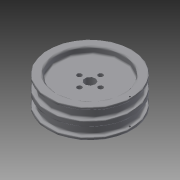
# Autodesk Inventor part: Spool
Saved by Autodesk Inventor 2014 SP2 (Build 180246200, 246)
## iProperties
Created: 2014-09-14
Part Number: Spool
Material: Generic
Document SubType Name: Modeling
Designer: Allison
Density: 1 g/cm^3
Appearance: Default
Author: Allison
Autodesk Inventor part; units mm, degrees
ref_plane "YZ Plane" through (0, 0, 0) normal (1, 0, 0) x (0, 1, 0)
ref_plane "XZ Plane" through (0, 0, 0) normal (0, 1, 0) x (-1, 0, 0)
ref_plane "XY Plane" through (0, 0, 0) normal (0, 0, 1) x (1, 0, 0)
sketch "Sketch1" plane through (0, 0, 0) normal (0, 1, 0) x (-1, 0, 0)
  circle A0 centre (0, 0) radius 31.75
  dimension "d0" = 63.5
  constraints: 1 centre point, 1 coincident
  measures "d0" diameter of A0
sketch "Sketch2" plane through (0, 0, 0) normal (1, 0, 0) x (0, 1, 0)
  line L0 (0, -31.75) -> (0, 31.75) projected
  line L1 (-3.6603, 0) -> (9.0397, 0)
  line L2 (9.0397, 0) -> (9.0397, 31.75)
  line L3 (-3.6603, 31.75) -> (-3.6603, 0)
  line L4 (-3.6603, 31.75) -> (-1.7553, 31.75)
  line L5 (-1.7553, 31.75) -> (-1.7553, 29.21)
  line L6 (9.0397, 31.75) -> (7.1347, 31.75)
  line L7 (7.1347, 31.75) -> (7.1347, 29.21)
  line L8 (7.1347, 29.21) -> (-1.7553, 29.21)
  line L9 (-3.6603, 0) -> (-3.6603, 4.0132)
  line L10 (-3.6603, 4.0132) -> (9.0397, 4.0132)
  line L11 (9.0397, 4.0132) -> (9.0397, 0)
  line L12 (9.0397, 0) -> (-3.6603, 0)
  line L13 (-3.6603, 0) -> (-3.6603, 4.0132)
  point P0 (0, 0)
  dimension "d1" = 12.7
  dimension "d2" = 1.905
  dimension "d5" = 1.905
  dimension "d6" = 31.75
  dimension "d7" = 4.0132
  constraints: 26 end point, 3 parallel, 2 horizontal, 2 perpendicular, 1 point on line
  measures "d1" distance of L3.start L2.end
  measures "d2" distance of L3.start L4.end
  measures "d5" distance of L2.end L6.end
  measures "d6" distance of L3.start L1.start
  measures "d7" distance of L1.start L9.end
revolve "Revolution1" add sketch "Sketch2" angle 360 about axis through (0, -3.6603, 0) along (0, 1, 0) contours L10 L3 L4 L5 L8 L0 | L0 L8 L7 L6 L2 L10
sketch "Sketch3" plane through (0, -3.6603, 0) normal (0, -1, 0) x (1, 0, 0)
  circle A0 centre (0, 0) radius 4.0132 projected
  circle A1 centre (0, 0) radius 31.75 projected
  line L0 (0, 0) -> (0, 8.001)
  circle A2 centre (0, 8.001) radius 1.8542
  circle A3 centre (-8.001, 0) radius 1.8542
  circle A4 centre (0, -8.001) radius 1.8542
  circle A5 centre (8.001, 0) radius 1.8542
  dimension "d10" = 8.001
  dimension "d11" = 3.7084
  dimension "d14" = 360
  constraints: 4 centre point, 2 end point, 1 coincident, 1 vertical, 9 other
  measures "d10" distance of L0.start L0.end
  measures "d11" diameter of A2
extrude "Extrusion1" cut sketch "Sketch3" against normal blind 25.4 contours A2 | A3 | A4 | A5
mirror "Mirror1" about plane through (0, 7.1347, 31.75) normal (0, -1, 0)
sketch "Sketch4" plane through (0, 17.9297, 0) normal (0, 1, 0) x (1, 0, 0)
  circle A0 centre (0, 8.001) radius 1.8542 projected
  circle A1 centre (0, -8.001) radius 1.8542 projected
  circle A2 centre (-8.001, 0) radius 1.8542 projected
  circle A3 centre (8.001, 0) radius 1.8542 projected
  circle A4 centre (0, 0) radius 4.0132 projected
  circle A5 centre (0, 0) radius 31.75 projected
  circle A6 centre (0, 0) radius 25.4
  dimension "d18" = 50.8
  constraints: 1 centre point, 1 coincident
  measures "d18" diameter of A6
extrude "Extrusion2" cut sketch "Sketch4" against normal blind 5.08 contours A6
fillet "Fillet2" radius 1.27 2 edges at (-25.4, 17.9297, 0) (-25.4, 12.8497, 0)
sketch "Sketch5" plane through (0, -3.6603, 0) normal (0, -1, 0) x (1, 0, 0)
  circle A0 centre (0, -8.001) radius 1.8542 projected
  circle A1 centre (0, 8.001) radius 1.8542 projected
  circle A2 centre (-8.001, 0) radius 1.8542 projected
  circle A3 centre (8.001, 0) radius 1.8542 projected
  circle A4 centre (0, 0) radius 4.0132 projected
  circle A5 centre (0, 0) radius 24.13 projected
  circle A6 centre (0, 0) radius 25.4
  dimension "d22" = 48.26
  dimension "d23" = 50.8
  constraints: 1 centre point, 1 coincident
  measures "d22" diameter of A5
  measures "d23" diameter of A6
extrude "Extrusion3" cut sketch "Sketch5" against normal blind 5.08 contours A5 | A6
fillet "Fillet3" radius 1.27 2 edges at (-25.4, -3.6603, 0) (-25.4, 1.4197, 0)
fillet "Fillet4" radius 0.508 6 edges at (0, -3.6603, -31.75) (0, -1.7553, -31.75) (0, 5.2297, -31.75) (0, 9.0397, -31.75) (0, 16.0247, -31.75) (0, 17.9297, -31.75)
sketch "Sketch6" plane through (0, -3.6603, 0) normal (0, -1, 0) x (1, 0, 0)
  circle A0 centre (0, 0) radius 29.21 projected
  circle A1 centre (30.2421, 0) radius 0.635
  dimension "d28" = 1.27
  constraints: 1 centre point
  measures "d28" diameter of A1
extrude "Extrusion4" cut sketch "Sketch6" against normal blind 7.62 contours A1
sketch "Sketch7" plane through (0, 17.9297, 0) normal (0, 1, 0) x (1, 0, 0)
  circle A0 centre (30.2421, 0) radius 0.635 projected
extrude "Extrusion5" cut sketch "Sketch7" against normal blind 7.62
fillet "Fillet5" radius 1.27 4 edges at (0, 16.0247, -29.21) (0, 9.0397, -29.21) (0, 5.2297, -29.21) (0, -1.7553, -29.21)
body "Solid1"
